Autodesk Inventor part; units mm, degrees
(part 2 of 2)
sketch "Sketch18" plane through (0, 0, 0) normal (0, -1, 0) x (1, 0, 0)
  circle A0 centre (63.2901, -137.289) radius 1.25 projected
  circle A1 centre (63.2901, -207.139) radius 1.25 projected
  line L0 (0, 0) -> (0, -56.6589)
  circle A2 centre (-48.2901, -137.289) radius 1.25
  circle A3 centre (-48.2901, -207.139) radius 1.25
  circle A4 centre (-48.2901, -137.289) radius 1.5
  circle A5 centre (-48.2901, -207.139) radius 1.5
  circle A6 centre (92.3731, -129.114) radius 1.25 projected
  circle A7 centre (76.8791, -129.114) radius 1.25 projected
  circle A8 centre (92.3731, -215.314) radius 1.25 projected
  circle A9 centre (76.8791, -215.314) radius 1.25 projected
  circle A10 centre (-48.2901, -207.139) radius 1.25
  circle A11 centre (-48.2901, -207.139) radius 1.5
  circle A12 centre (-77.3731, -129.114) radius 1.25
  circle A13 centre (-61.8791, -129.114) radius 1.25
  circle A14 centre (-77.3731, -215.314) radius 1.25
  circle A15 centre (-61.8791, -215.314) radius 1.25
  circle A16 centre (-77.3731, -215.314) radius 1.5
  circle A17 centre (-61.8791, -215.314) radius 1.5
  circle A18 centre (-77.3731, -129.114) radius 1.5
  circle A19 centre (-61.8791, -129.114) radius 1.5
  circle A20 centre (100.8821, -207.139) radius 1.25 projected
  circle A21 centre (100.8821, -137.289) radius 1.25 projected
  circle A22 centre (-48.2901, -207.139) radius 1.25
  circle A23 centre (-48.2901, -207.139) radius 1.5
  circle A24 centre (-77.3731, -129.114) radius 1.25
  circle A25 centre (-61.8791, -129.114) radius 1.25
  circle A26 centre (-77.3731, -215.314) radius 1.25
  circle A27 centre (-61.8791, -215.314) radius 1.25
  circle A28 centre (-77.3731, -215.314) radius 1.5
  circle A29 centre (-61.8791, -215.314) radius 1.5
  circle A30 centre (-77.3731, -129.114) radius 1.5
  circle A31 centre (-61.8791, -129.114) radius 1.5
  circle A32 centre (-85.8821, -207.139) radius 1.25
  circle A33 centre (-85.8821, -137.289) radius 1.25
  circle A34 centre (-85.8821, -207.139) radius 1.5
  circle A35 centre (-85.8821, -137.289) radius 1.5
  arc A36 (-149.2483, -194.3186) -> (-149.2483, -415.2814) centre (634.1788, -304.8) ccw projected
  line L1 (-157.0002, -304.8) -> (-226.6534, -304.8)
  line L2 (0, -609.6) -> (0, -552.9411)
  circle A37 centre (-48.2901, -472.311) radius 1.25
  circle A38 centre (-48.2901, -402.461) radius 1.25
  circle A39 centre (-48.2901, -472.311) radius 1.5
  circle A40 centre (-48.2901, -402.461) radius 1.5
  circle A41 centre (-48.2901, -402.461) radius 1.25
  circle A42 centre (-48.2901, -402.461) radius 1.5
  circle A43 centre (-61.8791, -394.286) radius 1.25
  circle A44 centre (-61.8791, -394.286) radius 1.5
  circle A45 centre (-77.3731, -394.286) radius 1.25
  circle A46 centre (-77.3731, -394.286) radius 1.5
  circle A47 centre (-48.2901, -472.311) radius 1.25
  circle A48 centre (-48.2901, -472.311) radius 1.5
  circle A49 centre (-61.8791, -480.486) radius 1.25
  circle A50 centre (-61.8791, -480.486) radius 1.5
  circle A51 centre (-77.3731, -480.486) radius 1.25
  circle A52 centre (-77.3731, -480.486) radius 1.5
  circle A53 centre (-48.2901, -402.461) radius 1.25
  circle A54 centre (-48.2901, -402.461) radius 1.5
  circle A55 centre (-85.8821, -402.461) radius 1.25
  circle A56 centre (-61.8791, -394.286) radius 1.25
  circle A57 centre (-61.8791, -394.286) radius 1.5
  circle A58 centre (-77.3731, -394.286) radius 1.25
  circle A59 centre (-77.3731, -394.286) radius 1.5
  circle A60 centre (-85.8821, -402.461) radius 1.5
  circle A61 centre (-85.8821, -472.311) radius 1.25
  circle A62 centre (-85.8821, -472.311) radius 1.5
  circle A63 centre (-48.2901, -472.311) radius 1.25
  circle A64 centre (-48.2901, -472.311) radius 1.5
  circle A65 centre (-77.3731, -480.486) radius 1.5
  circle A66 centre (-61.8791, -480.486) radius 1.25
  circle A67 centre (-61.8791, -480.486) radius 1.5
  circle A68 centre (-77.3731, -480.486) radius 1.25
  arc A69 (-149.2483, -194.3186) -> (-149.2483, -415.2814) centre (634.1788, -304.8) ccw
  line L3 (-63.2901, -137.289) -> (-48.2901, -137.289)
  circle A70 centre (48.2901, -137.289) radius 1.25
  circle A71 centre (48.2901, -207.139) radius 1.25
  circle A72 centre (48.2901, -137.289) radius 1.5
  circle A73 centre (48.2901, -207.139) radius 1.5
  circle A74 centre (48.2901, -207.139) radius 1.25
  circle A75 centre (48.2901, -207.139) radius 1.5
  circle A76 centre (61.8791, -215.314) radius 1.25
  circle A77 centre (61.8791, -215.314) radius 1.5
  circle A78 centre (77.3731, -215.314) radius 1.25
  circle A79 centre (77.3731, -215.314) radius 1.5
  circle A80 centre (61.8791, -129.114) radius 1.25
  circle A81 centre (61.8791, -129.114) radius 1.5
  circle A82 centre (77.3731, -129.114) radius 1.25
  circle A83 centre (77.3731, -129.114) radius 1.5
  circle A84 centre (48.2901, -207.139) radius 1.25
  circle A85 centre (48.2901, -207.139) radius 1.5
  circle A86 centre (85.8821, -207.139) radius 1.25
  circle A87 centre (61.8791, -215.314) radius 1.25
  circle A88 centre (61.8791, -215.314) radius 1.5
  circle A89 centre (77.3731, -215.314) radius 1.25
  circle A90 centre (77.3731, -215.314) radius 1.5
  circle A91 centre (85.8821, -207.139) radius 1.5
  circle A92 centre (85.8821, -137.289) radius 1.25
  circle A93 centre (85.8821, -137.289) radius 1.5
  circle A94 centre (77.3731, -129.114) radius 1.5
  circle A95 centre (61.8791, -129.114) radius 1.25
  circle A96 centre (61.8791, -129.114) radius 1.5
  circle A97 centre (77.3731, -129.114) radius 1.25
  circle A98 centre (48.2901, -472.311) radius 1.25
  circle A99 centre (48.2901, -402.461) radius 1.25
  circle A100 centre (48.2901, -472.311) radius 1.5
  circle A101 centre (48.2901, -402.461) radius 1.5
  circle A102 centre (48.2901, -472.311) radius 1.25
  circle A103 centre (48.2901, -472.311) radius 1.25
  circle A104 centre (48.2901, -472.311) radius 1.5
  circle A105 centre (48.2901, -472.311) radius 1.5
  circle A106 centre (48.2901, -402.461) radius 1.25
  circle A107 centre (48.2901, -402.461) radius 1.25
  circle A108 centre (48.2901, -402.461) radius 1.5
  circle A109 centre (48.2901, -402.461) radius 1.5
  circle A110 centre (61.8791, -480.486) radius 1.25
  circle A111 centre (61.8791, -480.486) radius 1.5
  circle A112 centre (77.3731, -480.486) radius 1.25
  circle A113 centre (77.3731, -480.486) radius 1.25
  circle A114 centre (77.3731, -480.486) radius 1.5
  circle A115 centre (61.8791, -480.486) radius 1.25
  circle A116 centre (61.8791, -480.486) radius 1.5
  circle A117 centre (77.3731, -480.486) radius 1.5
  circle A118 centre (61.8791, -394.286) radius 1.25
  circle A119 centre (61.8791, -394.286) radius 1.5
  circle A120 centre (77.3731, -394.286) radius 1.25
  circle A121 centre (77.3731, -394.286) radius 1.5
  circle A122 centre (85.8821, -472.311) radius 1.25
  circle A123 centre (85.8821, -472.311) radius 1.5
  circle A124 centre (61.8791, -394.286) radius 1.5
  circle A125 centre (61.8791, -394.286) radius 1.25
  circle A126 centre (85.8821, -402.461) radius 1.25
  circle A127 centre (85.8821, -402.461) radius 1.5
  circle A128 centre (77.3731, -394.286) radius 1.5
  circle A129 centre (77.3731, -394.286) radius 1.25
  line L4 (63.2901, -137.289) -> (48.2901, -137.289)
  dimension "d143" = 15
  constraints: 121 centre point, 66 symmetric about line, 60 coincident, 10 end point, 3 point on circle, 2 horizontal, 1 vertical, 61 other
  measures "d143" distance of L3.start L3.end
extrude "Extrusion24" cut sketch "Sketch18" against normal blind 10 contours A70 | A72 | A2 | A4 | A3 | A5 | A7 A82 | A7 A82 | A82 A7 A83 | A7 A83 A82 | A9 A78 | A9 A78 | A78 A9 A79 | A9 A79 A78 | A12 | A13 | A14 | A15 | A16 | A17 | A18 | A19 | A32 | A33 | A34 | A35 | A37 | A38 | A39 | A40 | A43 | A44 | A45 | A46 | A49 | A51 | A52 | A55 | A60 | A61 | A62 | A71 | A73 | A76 | A77 | A80 | A81 | A86 | A91 | A92 | A93 | A98 | A99 | A100 | A101 | A110 | A111 | A112 | A114 | A118 | A119 | A120 | A121 | A122 | A123 | A126 | A127
sketch "Sketch19" plane through (0, 0, 0) normal (0, -1, 0) x (1, 0, 0)
  line L0 (24.5, -126.055) -> (24.5, -171.055)
  arc A0 (24.5, -126.055) -> (20.5, -126.055) centre (22.5, -126.055) ccw
  line L1 (20.5, -171.055) -> (20.5, -126.055)
  arc A1 (20.5, -171.055) -> (24.5, -171.055) centre (22.5, -171.055) ccw
  line L2 (-20.5, -126.055) -> (-20.5, -171.055)
  line L3 (-24.5, -171.055) -> (-24.5, -126.055)
  arc A2 (-20.5, -126.055) -> (-24.5, -126.055) centre (-22.5, -126.055) ccw
  arc A3 (-24.5, -171.055) -> (-20.5, -171.055) centre (-22.5, -171.055) ccw
  line L4 (0, 0) -> (0, -305.0128)
  line L5 (23.3741, -126.055) -> (-21.6259, -126.055)
  line L6 (22.5, -171.055) -> (0, -171.055)
  point P0 (0, -171.055)
  point P1 (0.8741, -171.055)
  dimension "d147" = 45
  dimension "d148" = 22.5
  constraints: 14 end point, 8 point on circle, 4 centre point, 2 horizontal, 1 point on line, 1 vertical
  measures "d147" distance of L5.start L5.end
  measures "d148" distance of L6.start L6.end
extrude "Extrusion25" cut sketch "Sketch19" against normal blind 10 contours L2 A3 L3 A2 | L0 A1 L1 A0
sketch "Sketch20" plane through (0, 6.35, 0) normal (0, 1, 0) x (1, 0, 0)
  circle A0 centre (0.5994, 429.4598) radius 1.375
  circle A1 centre (0.5994, 429.4598) radius 1.63
  point P0 (0, 0)
  dimension "d161" = 3.26
  constraints: 2 centre point, 1 coincident, 2 other
  measures "d161" diameter of A1
extrude "Extrusion26" cut sketch "Sketch20" against normal blind 10 contours A0 | A1
sketch "Sketch21" plane through (0, 6.35, 0) normal (0, 1, 0) x (1, 0, 0)
  circle A0 centre (-57.1924, 314.2203) radius 1.625
  circle A1 centre (-57.1926, 304.2203) radius 1.625
  ellipse E0 centre (0, 304.8) end of major axis (0, 542.544) minor radius 177.8 (-124.461, 135.0182) -> (124.461, 135.0182) ccw projected
  line L0 (0, 304.8) -> (0, 359.0363)
  circle A2 centre (-57.1926, 304.2203) radius 1.75
  circle A3 centre (-57.1924, 314.2203) radius 1.75
  circle A4 centre (57.1924, 314.2203) radius 1.625
  circle A5 centre (57.1926, 304.2203) radius 1.625
  circle A6 centre (57.1926, 304.2203) radius 1.75
  circle A7 centre (57.1924, 314.2203) radius 1.75
  circle A8 centre (-57.1923, 329.8) radius 1.625
  circle A9 centre (-57.1923, 329.8) radius 1.625
  circle A10 centre (-57.1923, 329.8) radius 1.625
  circle A11 centre (-57.1923, 339.8) radius 1.625
  circle A12 centre (57.1924, 314.2203) radius 1.625
  circle A13 centre (57.1926, 304.2203) radius 1.625
  circle A14 centre (57.1924, 314.2203) radius 1.625
  circle A15 centre (57.1926, 304.2203) radius 1.625
  circle A16 centre (57.1927, 288.6407) radius 1.625
  circle A17 centre (57.1927, 278.6407) radius 1.625
  circle A18 centre (-57.1924, 314.2203) radius 1.625
  circle A19 centre (-57.1926, 304.2203) radius 1.625
  circle A20 centre (0.5994, 429.4598) radius 1.63 projected
  arc A21 (20.5, 126.055) -> (24.5, 126.055) centre (22.5, 126.055) ccw projected
  line L1 (24.5, 126.055) -> (24.5, 171.055) projected
  arc A22 (24.5, 171.055) -> (20.5, 171.055) centre (22.5, 171.055) ccw projected
  line L2 (20.5, 171.055) -> (20.5, 126.055) projected
  arc A23 (-24.5, 126.055) -> (-20.5, 126.055) centre (-22.5, 126.055) ccw projected
  line L3 (-20.5, 126.055) -> (-20.5, 171.055) projected
  arc A24 (-20.5, 171.055) -> (-24.5, 171.055) centre (-22.5, 171.055) ccw projected
  line L4 (-24.5, 171.055) -> (-24.5, 126.055) projected
  circle A25 centre (-61.8791, 480.486) radius 1.25 projected
  circle A26 centre (77.3731, 215.314) radius 1.5 projected
  circle A27 centre (85.8821, 402.461) radius 1.5 projected
  circle A28 centre (77.3731, 480.486) radius 1.5 projected
  circle A29 centre (61.8791, 394.286) radius 1.5 projected
  circle A30 centre (48.2901, 472.311) radius 1.5 projected
  circle A31 centre (61.8791, 129.114) radius 1.5 projected
  circle A32 centre (61.8791, 215.314) radius 1.5 projected
  circle A33 centre (48.2901, 137.289) radius 1.5 projected
  circle A34 centre (-85.8821, 472.311) radius 1.5 projected
  circle A35 centre (-61.8791, 394.286) radius 1.5 projected
  circle A36 centre (-48.2901, 402.461) radius 1.5 projected
  circle A37 centre (-85.8821, 137.289) radius 1.5 projected
  circle A38 centre (-77.3731, 129.114) radius 1.5 projected
  circle A39 centre (-77.3731, 215.314) radius 1.5 projected
  circle A40 centre (-48.2901, 207.139) radius 1.5 projected
  circle A41 centre (-48.2901, 137.289) radius 1.5 projected
  circle A42 centre (-61.8791, 215.314) radius 1.5 projected
  circle A43 centre (-61.8791, 129.114) radius 1.5 projected
  circle A44 centre (-85.8821, 207.139) radius 1.5 projected
  circle A45 centre (-48.2901, 472.311) radius 1.5 projected
  circle A46 centre (-77.3731, 480.486) radius 1.5 projected
  circle A47 centre (-77.3731, 394.286) radius 1.5 projected
  circle A48 centre (-85.8821, 402.461) radius 1.5 projected
  circle A49 centre (48.2901, 207.139) radius 1.5 projected
  circle A50 centre (85.8821, 207.139) radius 1.5 projected
  circle A51 centre (85.8821, 137.289) radius 1.5 projected
  circle A52 centre (77.3731, 394.286) radius 1.5 projected
  circle A53 centre (61.8791, 480.486) radius 1.5 projected
  circle A54 centre (85.8821, 472.311) radius 1.5 projected
  circle A55 centre (48.2901, 402.461) radius 1.5 projected
  circle A56 centre (77.3731, 129.114) radius 1.5 projected
  arc A57 (-149.2483, 194.3186) -> (-124.461, 135.0182) centre (-23.4926, 212.0531) ccw projected
  arc A58 (-149.2483, 415.2814) -> (-149.2483, 194.3186) centre (634.1788, 304.8) ccw projected
  arc A59 (-124.461, 474.5818) -> (-149.2483, 415.2814) centre (-23.4926, 397.5469) ccw projected
  ellipse E1 centre (0, 304.8) end of major axis (0, 542.544) minor radius 177.8 (124.461, 474.5818) -> (-124.461, 474.5818) ccw projected
  arc A60 (149.2483, 415.2814) -> (124.461, 474.5818) centre (23.4926, 397.5469) ccw projected
  arc A61 (149.2483, 194.3186) -> (149.2483, 415.2814) centre (-634.1788, 304.8) ccw projected
  arc A62 (124.461, 135.0182) -> (149.2483, 194.3186) centre (23.4926, 212.0531) ccw projected
  ellipse E2 centre (0, 304.8) end of major axis (0, 542.544) minor radius 177.8 (-124.461, 135.0182) -> (124.461, 135.0182) ccw projected
  line L5 (59.3547, 229.7811) -> (63.3547, 229.7811) projected
  arc A63 (63.3547, 229.7811) -> (63.3547, 232.7809) centre (63.3547, 231.281) ccw projected
  line L6 (63.3547, 232.7809) -> (59.3547, 232.7809) projected
  arc A64 (59.3547, 232.7809) -> (59.3547, 229.7811) centre (59.3547, 231.281) ccw projected
  line L7 (59.3087, 294.4643) -> (63.3087, 294.4643) projected
  arc A65 (63.3087, 294.4643) -> (63.3087, 297.4641) centre (63.3087, 295.9642) ccw projected
  line L8 (63.3087, 297.4641) -> (59.3087, 297.4641) projected
  arc A66 (59.3087, 297.4641) -> (59.3087, 294.4643) centre (59.3087, 295.9642) ccw projected
  line L9 (-55.1482, 229.6998) -> (-51.1482, 229.6998) projected
  arc A67 (-51.1482, 229.6998) -> (-51.1482, 232.6996) centre (-51.1482, 231.1997) ccw projected
  line L10 (-51.1482, 232.6996) -> (-55.1482, 232.6996) projected
  arc A68 (-55.1482, 232.6996) -> (-55.1482, 229.6998) centre (-55.1482, 231.1997) ccw projected
  line L11 (-55.1942, 294.4643) -> (-51.1942, 294.4643) projected
  arc A69 (-51.1942, 294.4643) -> (-51.1942, 297.4641) centre (-51.1942, 295.9642) ccw projected
  line L12 (-51.1942, 297.4641) -> (-55.1942, 297.4641) projected
  arc A70 (-55.1942, 297.4641) -> (-55.1942, 294.4643) centre (-55.1942, 295.9642) ccw projected
  arc A71 (30.8456, 314.5355) -> (33.8432, 314.5354) centre (32.3444, 314.5355) ccw projected
  line L13 (33.8432, 314.5354) -> (33.8433, 318.5354) projected
  arc A72 (33.8433, 318.5354) -> (30.8454, 318.5354) centre (32.3444, 318.5355) ccw projected
  line L14 (30.8454, 318.5354) -> (30.8456, 314.5355) projected
  arc A73 (30.9268, 200.0992) -> (33.9251, 200.144) centre (32.4256, 200.1453) ccw projected
  line L15 (33.9251, 200.144) -> (33.9246, 204.1455) projected
  arc A74 (33.9246, 204.1455) -> (30.9266, 204.1452) centre (32.4256, 204.1453) ccw projected
  line L16 (30.9266, 204.1452) -> (30.9268, 200.0992) projected
  line L17 (-33.9248, 211.7492) -> (-33.9246, 207.7493) projected
  arc A75 (-33.9246, 207.7493) -> (-30.927, 207.7491) centre (-32.4258, 207.7492) ccw projected
  line L18 (-30.927, 207.7491) -> (-30.9268, 211.7491) projected
  arc A76 (-30.9268, 211.7491) -> (-33.9248, 211.7492) centre (-32.4258, 211.7492) ccw projected
  arc A77 (30.8401, 322.1854) -> (33.8377, 322.1855) centre (32.3389, 322.1855) ccw projected
  line L19 (33.8377, 322.1855) -> (33.8379, 326.1854) projected
  arc A78 (33.8379, 326.1854) -> (30.8399, 326.1854) centre (32.3389, 326.1855) ccw projected
  line L20 (30.8399, 326.1854) -> (30.8401, 322.1854) projected
  circle A79 centre (27.1519, 360.7012) radius 1.25 projected
  circle A80 centre (-21.8701, 360.917) radius 1.25 projected
  circle A81 centre (-31.3951, 388.1966) radius 1.25 projected
  circle A82 centre (-31.3951, 412.3128) radius 1.25 projected
  circle A83 centre (-21.8701, 415.4878) radius 1.25 projected
  circle A84 centre (-31.3951, 364.092) radius 1.25 projected
  circle A85 centre (27.1519, 405.5552) radius 1.25 projected
  arc A86 (30.9214, 207.7522) -> (33.919, 207.7521) centre (32.4202, 207.7522) ccw projected
  line L21 (33.919, 207.7521) -> (33.9192, 211.7521) projected
  arc A87 (33.9192, 211.7521) -> (30.9212, 211.7521) centre (32.4202, 211.7522) ccw projected
  line L22 (30.9212, 211.7521) -> (30.9214, 207.7522) projected
  arc A88 (-33.9299, 322.1395) -> (-30.9323, 322.1395) centre (-32.4311, 322.1395) ccw projected
  line L23 (-30.9323, 322.1395) -> (-30.9321, 326.1394) projected
  arc A89 (-30.9321, 326.1394) -> (-33.93, 326.1394) centre (-32.4311, 326.1395) ccw projected
  line L24 (-33.93, 326.1394) -> (-33.9299, 322.1395) projected
  arc A90 (-33.9246, 200.0993) -> (-30.927, 200.0992) centre (-32.4258, 200.0993) ccw projected
  line L25 (-30.927, 200.0992) -> (-30.9268, 204.0992) projected
  arc A91 (-30.9268, 204.0992) -> (-33.9248, 204.0992) centre (-32.4258, 204.0993) ccw projected
  line L26 (-33.9248, 204.0992) -> (-33.9246, 200.0993) projected
  arc A92 (-33.9295, 314.4894) -> (-30.9319, 314.4894) centre (-32.4307, 314.4895) ccw projected
  line L27 (-30.9319, 314.4894) -> (-30.9317, 318.4894) projected
  arc A93 (-30.9317, 318.4894) -> (-33.9297, 318.4894) centre (-32.4307, 318.4895) ccw projected
  line L28 (-33.9297, 318.4894) -> (-33.9295, 314.4894) projected
  line L29 (-58.8442, 297.4645) -> (-62.8442, 297.4645) projected
  arc A94 (-62.8442, 297.4645) -> (-62.8442, 294.4646) centre (-62.8442, 295.9646) ccw projected
  line L30 (-62.8442, 294.4646) -> (-58.8442, 294.4646) projected
  arc A95 (-58.8442, 294.4646) -> (-58.8442, 297.4645) centre (-58.8442, 295.9646) ccw projected
  line L31 (-62.8442, 229.6943) -> (-58.8442, 229.6943) projected
  arc A96 (-58.8442, 229.6943) -> (-58.8442, 232.6942) centre (-58.8442, 231.1942) ccw projected
  line L32 (-58.8442, 232.6942) -> (-62.8442, 232.6942) projected
  arc A97 (-62.8442, 232.6942) -> (-62.8442, 229.6943) centre (-62.8442, 231.1942) ccw projected
  line L33 (51.6587, 294.4643) -> (55.6587, 294.4643) projected
  arc A98 (55.6587, 294.4643) -> (55.6587, 297.4641) centre (55.6587, 295.9642) ccw projected
  line L34 (55.6587, 297.4641) -> (51.6587, 297.4641) projected
  arc A99 (51.6587, 297.4641) -> (51.6587, 294.4643) centre (51.6587, 295.9642) ccw projected
  line L35 (51.7047, 229.7757) -> (55.7047, 229.7757) projected
  arc A100 (55.7047, 229.7757) -> (55.7047, 232.7755) centre (55.7047, 231.2756) ccw projected
  line L36 (55.7047, 232.7755) -> (51.7047, 232.7755) projected
  arc A101 (51.7047, 232.7755) -> (51.7047, 229.7757) centre (51.7047, 231.2756) ccw projected
  circle A102 centre (0, 263.5227) radius 35 projected
  line L37 (14.9599, 357.742) -> (14.9599, 418.6628) projected
  line L38 (14.9599, 418.6628) -> (-15.5201, 418.6628) projected
  line L39 (-15.5201, 418.6628) -> (-15.5201, 357.742) projected
  line L40 (-15.5201, 357.742) -> (14.9599, 357.742) projected
  circle A103 centre (-11.1, 511.544) radius 1.5 projected
  circle A104 centre (11.1, 511.544) radius 1.5 projected
  circle A105 centre (9.275, 529.719) radius 1.5 projected
  circle A106 centre (17.082, 448.0427) radius 1.5 projected
  circle A107 centre (24.257, 455.2177) radius 1.5 projected
  circle A108 centre (-14.097, 455.2177) radius 1.5 projected
  circle A109 centre (-6.922, 448.0427) radius 1.5 projected
  circle A110 centre (-9.275, 529.719) radius 1.5 projected
  circle A111 centre (11.1, 519.544) radius 1.5 projected
  circle A112 centre (-11.1, 519.544) radius 1.5 projected
  circle A113 centre (-32.3895, 82.38) radius 1.25 projected
  circle A114 centre (32.3895, 152.23) radius 1.25 projected
  circle A115 centre (32.3895, 82.38) radius 1.25 projected
  circle A116 centre (-32.3895, 152.23) radius 1.25 projected
  circle A117 centre (57.1928, 329.8) radius 1.625
  circle A118 centre (57.1928, 339.8) radius 1.625
  circle A119 centre (-57.1923, 329.8) radius 1.75
  circle A120 centre (-57.1923, 339.8) radius 1.75
  circle A121 centre (57.1928, 329.8) radius 1.75
  circle A122 centre (57.1928, 339.8) radius 1.75
  point P0 (0, 0)
  dimension "d164" = 3.5
  dimension "d165" = 3.5
  dimension "d168" = 3.5
  dimension "d169" = 3.5
  dimension "d170" = 3.5
  dimension "d171" = 3.5
  constraints: 26 centre point, 8 coincident, 4 symmetric about line, 2 end point, 1 vertical, 39 other
  measures "d164" diameter of A2
  measures "d165" diameter of A3
  measures "d168" diameter of A119
  measures "d169" diameter of A120
  measures "d170" diameter of A121
  measures "d171" diameter of A122
extrude "Extrusion27" cut sketch "Sketch21" against normal blind 10 contours A0 | A1 | A2 | A3 | A4 | A5 | A6 | A7 | A8 | A11 | A117 | A118 | A119 | A120 | A121 | A122
sketch "Sketch22" plane through (0, 6.35, 0) normal (0, 1, 0) x (1, 0, 0)
  circle A0 centre (-69.1987, 381.8) radius 1.625
  circle A1 centre (-54.3387, 381.8) radius 1.625
  circle A2 centre (-54.3387, 349.8) radius 1.625
  circle A3 centre (-69.1987, 349.8) radius 1.625
  circle A4 centre (-69.1987, 349.8) radius 1.75
  circle A5 centre (-54.3387, 349.8) radius 1.75
  circle A6 centre (-69.1987, 381.8) radius 1.75
  circle A7 centre (-54.3387, 381.8) radius 1.75
  point P0 (0, 0)
  dimension "d172" = 3.5
  dimension "d173" = 3.5
  dimension "d174" = 3.5
  dimension "d175" = 3.5
  constraints: 8 centre point, 4 coincident, 8 other
  measures "d172" diameter of A4
  measures "d173" diameter of A5
  measures "d174" diameter of A6
  measures "d175" diameter of A7
extrude "Extrusion28" [suppressed]
sketch "Sketch23" plane through (0, 6.35, 0) normal (0, 1, 0) x (1, 0, 0)
  circle A0 centre (-83.3424, 232.0248) radius 1.625
  circle A1 centre (-83.3424, 264.0248) radius 1.625
  circle A2 centre (-98.2024, 264.0248) radius 1.625
  circle A3 centre (-98.2024, 232.0248) radius 1.625
  circle A4 centre (-98.2024, 232.0248) radius 1.75
  circle A5 centre (-83.3424, 232.0248) radius 1.75
  circle A6 centre (-98.2024, 264.0248) radius 1.75
  circle A7 centre (-83.3424, 264.0248) radius 1.75
  circle A8 centre (-124.3469, 231.8724) radius 1.5
  circle A9 centre (-124.3469, 274.5248) radius 1.5
  circle A10 centre (-124.3469, 231.8724) radius 1.75
  circle A11 centre (-124.3469, 274.5248) radius 1.75
  line L0 (0, -1.4323) -> (0, -87.4076)
  circle A12 centre (83.3424, 232.0248) radius 1.625
  circle A13 centre (83.3424, 264.0248) radius 1.625
  circle A14 centre (98.2024, 264.0248) radius 1.625
  circle A15 centre (98.2024, 232.0248) radius 1.625
  circle A16 centre (98.2024, 232.0248) radius 1.75
  circle A17 centre (83.3424, 232.0248) radius 1.75
  circle A18 centre (98.2024, 264.0248) radius 1.75
  circle A19 centre (83.3424, 264.0248) radius 1.75
  circle A20 centre (124.3469, 231.8724) radius 1.5
  circle A21 centre (124.3469, 274.5248) radius 1.5
  circle A22 centre (124.3469, 231.8724) radius 1.75
  circle A23 centre (124.3469, 274.5248) radius 1.75
  point P0 (0, 0)
  dimension "d178" = 3.5
  dimension "d179" = 3.5
  dimension "d180" = 3.5
  dimension "d181" = 3.5
  dimension "d184" = 3.5
  dimension "d185" = 3.5
  constraints: 24 centre point, 12 coincident, 12 symmetric about line, 2 end point, 1 vertical, 24 other
  measures "d178" diameter of A4
  measures "d179" diameter of A5
  measures "d180" diameter of A6
  measures "d181" diameter of A7
  measures "d184" diameter of A10
  measures "d185" diameter of A11
extrude "Extrusion29" cut sketch "Sketch23" against normal blind 10 contours A0 | A1 | A2 | A3 | A4 | A5 | A6 | A7 | A8 | A9 | A10 | A11 | A12 | A13 | A14 | A15 | A16 | A17 | A18 | A19 | A20 | A21 | A22 | A23
sketch "Sketch24" plane through (0, 6.35, 0) normal (0, 1, 0) x (1, 0, 0)
  circle A0 centre (-93.4574, 331.6674) radius 1.5
  circle A1 centre (-99.6613, 341.1674) radius 1.5
  circle A2 centre (-93.4574, 351.8794) radius 1.5
  circle A3 centre (-99.6613, 362.5914) radius 1.5
  circle A4 centre (-93.4574, 372.0914) radius 1.5
  line L0 (-105.0574, 309.5458) -> (-105.0574, 383.1458)
  line L1 (-115.8574, 309.5458) -> (-115.8574, 383.1458)
  line L2 (-122.3207, 309.5458) -> (-99.5255, 309.5458)
  line L3 (-110.9231, 309.5458) -> (-110.9231, 321.5085)
  circle A5 centre (-93.4574, 331.6674) radius 1.75
  circle A6 centre (-99.6613, 341.1674) radius 1.75
  circle A7 centre (-93.4574, 351.8794) radius 1.75
  circle A8 centre (-99.6613, 362.5914) radius 1.75
  circle A9 centre (-93.4574, 372.0914) radius 1.75
  circle A10 centre (-128.3888, 331.6674) radius 1.5
  circle A11 centre (-122.1849, 341.1674) radius 1.5
  circle A12 centre (-128.3888, 351.8794) radius 1.5
  circle A13 centre (-122.1849, 362.5914) radius 1.5
  circle A14 centre (-128.3888, 372.0914) radius 1.5
  circle A15 centre (-128.3888, 331.6674) radius 1.75
  circle A16 centre (-122.1849, 341.1674) radius 1.75
  circle A17 centre (-128.3888, 351.8794) radius 1.75
  circle A18 centre (-122.1849, 362.5914) radius 1.75
  circle A19 centre (-128.3888, 372.0914) radius 1.75
  line L4 (0, 0) -> (0, 23.2799)
  circle A20 centre (93.4574, 331.6674) radius 1.5
  circle A21 centre (99.6613, 341.1674) radius 1.5
  circle A22 centre (93.4574, 351.8794) radius 1.5
  circle A23 centre (99.6613, 362.5914) radius 1.5
  circle A24 centre (93.4574, 372.0914) radius 1.5
  line L5 (105.0574, 309.5458) -> (105.0574, 383.1458)
  line L6 (115.8574, 309.5458) -> (115.8574, 383.1458)
  line L7 (122.3207, 309.5458) -> (99.5255, 309.5458)
  line L8 (110.9231, 309.5458) -> (110.9231, 321.5085)
  circle A25 centre (93.4574, 331.6674) radius 1.75
  circle A26 centre (99.6613, 341.1674) radius 1.75
  circle A27 centre (93.4574, 351.8794) radius 1.75
  circle A28 centre (99.6613, 362.5914) radius 1.75
  circle A29 centre (93.4574, 372.0914) radius 1.75
  circle A30 centre (122.1849, 362.5914) radius 1.75
  circle A31 centre (128.3888, 351.8794) radius 1.5
  circle A32 centre (128.3888, 351.8794) radius 1.75
  circle A33 centre (128.3888, 372.0914) radius 1.5
  circle A34 centre (128.3888, 372.0914) radius 1.75
  circle A35 centre (122.1849, 341.1674) radius 1.5
  circle A36 centre (122.1849, 341.1674) radius 1.75
  circle A37 centre (128.3888, 331.6674) radius 1.5
  circle A38 centre (128.3888, 331.6674) radius 1.75
  circle A39 centre (122.1849, 362.5914) radius 1.5
  dimension "d186" = 3.5
  dimension "d187" = 3.5
  dimension "d188" = 3.5
  dimension "d189" = 3.5
  dimension "d190" = 3.5
  constraints: 40 centre point, 38 symmetric about line, 20 coincident, 18 end point, 4 vertical, 1 horizontal, 1 midpoint, 46 other
  measures "d186" diameter of A5
  measures "d187" diameter of A6
  measures "d188" diameter of A7
  measures "d189" diameter of A8
  measures "d190" diameter of A9
extrude "Extrusion30" cut sketch "Sketch24" against normal blind 10 contours A0 | A1 | A2 | A3 | A4 | A5 | A6 | A7 | A8 | A9 | A10 | A11 | A12 | A13 | A14 | A15 | A16 | A17 | A18 | A19 | A20 | A21 | A22 | A23 | A24 | A25 | A26 | A27 | A28 | A29 | A30 | A31 | A32 | A33 | A34 | A35 | A36 | A37 | A38 | A39
body "Solid2"
